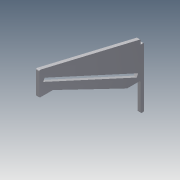
# Autodesk Inventor part: ControlRightPanel
Saved by Autodesk Inventor 2014 (Build 180170000, 170)
## iProperties
Created: 2015-01-19
Part Number: ControlRightPanel
Material: Generic
Document SubType Name: Modeling
Designer: Peele
Density: 1 g/cm^3
Appearance: White
Author: Peele
Autodesk Inventor part; units mm, degrees
ref_plane "YZ Plane" through (0, 0, 0) normal (1, 0, 0) x (0, 1, 0)
ref_plane "XZ Plane" through (0, 0, 0) normal (0, 1, 0) x (-1, 0, 0)
ref_plane "XY Plane" through (0, 0, 0) normal (0, 0, 1) x (1, 0, 0)
sketch "Sketch1" plane through (0, 0, 0) normal (1, 0, 0) x (0, 1, 0)
  line L0 (0, 0) -> (0, 25) construction
  line L1 (185, -25) -> (185, -90)
  line L2 (185, -25) -> (-25, 25) construction
  line L3 (0, 0) -> (0, 19.0476)
  line L4 (0, 19.0476) -> (185, -25)
  line L5 (0, -25) -> (0, 0)
  line L6 (185, -90) -> (160, -90)
  line L7 (0, -25) -> (25, -25)
  line L8 (25, -25) -> (160, -90)
  dimension "d0" = 25
  dimension "d1" = 65
  dimension "d2" = 185
  dimension "d10" = 25
  dimension "d11" = 25
  dimension "d17" = 25
  dimension "d20" = 25
  constraints: 18 end point, 3 parallel, 2 point on line, 1 collinear, 1 horizontal alignment, 1 perpendicular, 1 vertical
  measures "d0" distance of L0.start L0.end
  measures "d1" distance of L1.start L1.end
  measures "d2" distance between parallel lines of L0 L1
  measures "d10" vertical distance of L0.start L1.start
  measures "d11" distance from line of L2.end L0
  measures "d17" distance of L5.start L0.start
  measures "d20" distance of L1.end L6.end
extrude "Extrusion1" add sketch "Sketch1" along normal blind 6
sketch "Sketch3" plane through (6, 0, 0) normal (1, 0, 0) x (0, 0, -1)
  line L0 (90, 185) -> (25, 185) projected
  line L1 (33.1, 185) -> (141.9, 185)
  line L2 (141.9, 185) -> (141.9, 191)
  line L3 (141.9, 191) -> (33.1, 191)
  line L4 (33.1, 191) -> (33.1, 185)
  dimension "d12" = 8.1
  dimension "d14" = 6
  dimension "d21" = 108.8
  constraints: 8 end point, 2 parallel, 1 horizontal, 1 perpendicular, 1 point on line
  measures "d12" distance from line of L0.end L4
  measures "d14" distance of L1.end L2.end
  measures "d21" distance of L2.end L3.end
extrude "Extrusion3" add sketch "Sketch3" against normal blind 6
sketch "Sketch4" plane through (6, 0, 0) normal (1, 0, 0) x (0, 0, -1)
  line L0 (0, 0) -> (85, 185) construction
  line L1 (3.34, 7.2694) -> (-2.1121, 9.7744)
  line L2 (-2.1121, 9.7744) -> (76.2079, 180.2356)
  line L3 (76.2079, 180.2356) -> (81.66, 177.7306)
  line L4 (3.34, 7.2694) -> (81.66, 177.7306)
  dimension "d23" = 185
  dimension "d24" = 85
  dimension "d28" = 8
  dimension "d29" = 8
  dimension "d32" = 6
  constraints: 10 end point, 3 perpendicular, 2 point on line, 1 parallel
  measures "d23" vertical distance of L0.start L0.end
  measures "d24" horizontal distance of L0.start L0.end
  measures "d28" distance from line of L0.start L1
  measures "d29" distance from line of L0.end L3
  measures "d32" distance between parallel lines of L2 L4
extrude "Extrusion4" cut sketch "Sketch4" against normal through all
fillet "Fillet1" radius 2 9 edges at (3, 185, -25) (3, 191, -33.1) (3, 191, -141.9) (3, 185, -141.9) (3, 185, -90) (3, 160, -90) (3, 25, -25) (3, 0, -25) (3, 0, 19.0476)
body "Solid1"
